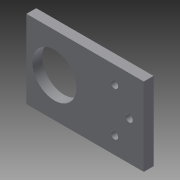
# Autodesk Inventor part: Light Bracket
Saved by Autodesk Inventor 2014 (Build 180170000, 170)
## iProperties
Created: 2014-02-12
Part Number: Light Bracket
Material: Generic
Document SubType Name: Sheet Metal
Designer: 2014180
Density: 1 g/cm^3
Sheet Metal Rule: Default
Appearance: Default
Author: 2014180
Autodesk Inventor part; units mm, degrees
ref_plane "YZ Plane" through (0, 0, 0) normal (1, 0, 0) x (0, 1, 0)
ref_plane "XZ Plane" through (0, 0, 0) normal (0, 1, 0) x (-1, 0, 0)
ref_plane "XY Plane" through (0, 0, 0) normal (0, 0, 1) x (1, 0, 0)
sketch "Sketch1" plane through (0, 0, 0) normal (0, 0, 1) x (1, 0, 0)
  line L0 (0, 0) -> (76.2, 0)
  line L1 (76.2, 0) -> (76.2, 50.8)
  line L2 (76.2, 50.8) -> (0, 50.8)
  line L3 (0, 50.8) -> (0, 0)
  circle A0 centre (18.1795, 25.4) radius 14.2875
  line L4 (76.2, 50.8) -> (57.15, 50.8)
  line L5 (57.15, 39.6875) -> (66.675, 25.4)
  line L6 (66.675, 25.4) -> (57.15, 11.1125)
  dimension "d0" = 76.2
  dimension "d1" = 50.8
  dimension "d2" = 28.575
  constraints: 14 end point, 2 parallel, 1 centre point, 1 horizontal, 1 perpendicular, 1 point on line
  measures "d0" distance of L2.end L1.end
  measures "d1" distance of L1.end L0.end
  measures "d2" diameter of A0
extrude "Extrusion1" add sketch "Sketch1" along normal blind 6.35
sketch "Sketch2" plane through (0, 0, 6.35) normal (0, 0, 1) x (1, 0, 0)
  line L0 (76.2, 50.8) -> (0, 50.8) projected
  line L1 (76.2, 50.8) -> (57.15, 50.8)
  line L2 (57.15, 39.6875) -> (66.675, 25.4)
  line L3 (66.675, 25.4) -> (57.15, 11.1125)
  constraints: 6 end point, 1 point on line
hole "Hole1" at (66.675, 25.4, 6.35) at (57.15, 39.6875, 6.35) at (57.15, 11.1125, 6.35) direction (0, 0, -1) diameter 4.7625 end through all
equation "\"d12\" = Thickness"
equation "\"BendRadius\" = Thickness"
equation "\"BendReliefWidth\" = Thickness"
equation "\"BendReliefDepth\" = 0.5 * Thickness"
equation "\"CornerReliefSize\" = 4 * Thickness"
equation "\"MinimumRemnant\" = 2 * Thickness"
equation "\"TransitionRadius\" = BendRadius"
equation "\"JacobiRadiusSize\" = BendRadius"
equation "\"GapSize\" = Thickness"
equation "\"Thickness\" = 3.048"
body "Solid1"
